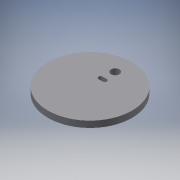
# Autodesk Inventor part: Aft Endcap Outer
Saved by Autodesk Inventor 2016 (Build 200138000, 138)
## iProperties
Created: 2015-06-17
Part Number: Aft Endcap Outer
Material: Generic
Document SubType Name: Modeling
Designer: JR
Density: 1 g/cm^3
Appearance: Default
Author: JR
Autodesk Inventor part; units mm, degrees
ref_plane "YZ Plane" through (0, 0, 0) normal (1, 0, 0) x (0, 1, 0)
ref_plane "XZ Plane" through (0, 0, 0) normal (0, 1, 0) x (-1, 0, 0)
ref_plane "XY Plane" through (0, 0, 0) normal (0, 0, 1) x (1, 0, 0)
sketch "Sketch1" plane through (0, 0, 0) normal (0, 0, 1) x (1, 0, 0)
  circle A0 centre (0, 0) radius 20
  line L0 (-1, 7) -> (1, 7)
  line L1 (1, 5) -> (-1, 5)
  circle A1 centre (0, 12) radius 2
  arc A2 (-1, 7) -> (-2, 6) centre (-1, 6) ccw
  arc A3 (-2, 6) -> (-1, 5) centre (-1, 6) ccw
  arc A4 (2, 6) -> (1, 7) centre (1, 6) ccw
  arc A5 (1, 5) -> (2, 6) centre (1, 6) ccw
  point P0 (-2, 7)
  point P1 (2, 5)
  point P2 (-2, 5)
  point P3 (0, 7)
  point P4 (0, 5)
  dimension "d0" = 40
  dimension "d1" = 4
  dimension "d2" = 4
  dimension "d3" = 2
  dimension "d4" = 1
  dimension "d5" = 12
  dimension "d6" = 5
  constraints: 8 point on circle, 6 centre point, 4 end point, 4 tangent, 3 point on line, 2 equal radius, 2 horizontal, 2 midpoint, 2 vertical alignment, 1 coincident, 1 concentric, 1 parallel, 13 other
  measures "d0" diameter of A0
  measures "d1" diameter of A1
  measures "d2" distance of point (2, 5) point (-2, 5)
  measures "d3" distance of point (-2, 5) point (-2, 7)
  measures "d4" radius of A2
  measures "d5" distance of point (0, 0) A1.centre
  measures "d6" distance from line of point (0, 0) L1
extrude "Extrusion1" add sketch "Sketch1" along normal blind 3
equation "\"d0\" = BattECOD"
equation "\"BattECOD\" = 40"
body "Solid1"
